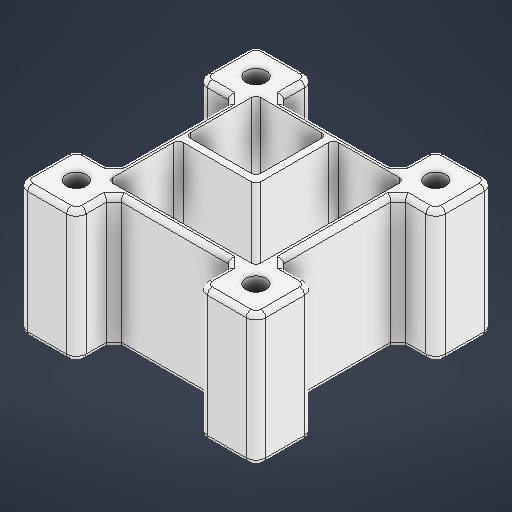
# Autodesk Inventor part: SemillasyAgua
Saved by Autodesk Inventor 2026.2 (Build 302298000, 298)
## iProperties
Created: 2025-11-15
Part Number: SemillasyAgua
Material: PLA
Document SubType Name: Modeling
Designer: vickh
Density: 1.3 g/cm^3
Appearance: Genérico
Mass: 211.053 g
Surface Area: 621.893 cm^2
Volume: 162.348 cm^3
Author: vickh
## iProperties of the stored document SemillasyAgua_3DPrint.ipt
Created: 2025-11-18
Part Number: SemillasyAgua_3DPrint
Material: Genérico
Document SubType Name: Modeling
Designer: usuario
Density: 1 g/cm^3
Appearance: Valor por defecto
Author: usuario
Autodesk Inventor part; units mm, degrees
ref_plane "YZ Plane" through (0, 0, 0) normal (1, 0, 0) x (0, 1, 0)
ref_plane "XZ Plane" through (0, 0, 0) normal (0, 1, 0) x (-1, 0, 0)
ref_plane "XY Plane" through (0, 0, 0) normal (0, 0, 1) x (1, 0, 0)
sketch "Boceto1" plane through (0, 0, 0) normal (0, 1, 0) x (-1, 0, 0)
  line L0 (25, 33.5) -> (-25, 33.5)
  line L1 (33.5, -25) -> (33.5, 25)
  circle A0 centre (0, 0) radius 5 construction
  line L2 (-33.5, 25) -> (-33.5, -25)
  line L3 (-25, -33.5) -> (25, -33.5)
  line L4 (-25, -49) -> (-25, -33.5)
  line L5 (-33.5, -25) -> (-49, -25)
  line L6 (-49, -25) -> (-49, -49)
  line L7 (-49, -49) -> (-25, -49)
  line L8 (-49, 25) -> (-33.5, 25)
  line L9 (-49, 49) -> (-49, 25)
  line L10 (-25, 49) -> (-49, 49)
  line L11 (-25, 33.5) -> (-25, 49)
  line L12 (33.5, 25) -> (49, 25)
  circle A1 centre (37, 37) radius 4.15
  line L13 (49, 25) -> (49, 49)
  line L14 (49, 49) -> (25, 49)
  line L15 (25, 49) -> (25, 33.5)
  line L16 (49, -49) -> (49, -25)
  line L17 (49, -25) -> (33.5, -25)
  line L18 (25, -49) -> (49, -49)
  line L19 (25, -33.5) -> (25, -49)
  line L20 (49, -49) -> (-49, -49) construction
  line L21 (-49, -49) -> (-49, 49)
  line L22 (-49, 49) -> (49, 49) construction
  line L23 (49, 49) -> (49, -49) construction
  line L24 (49, -49) -> (15.5795, -49) construction
  line L25 (49, -27.4055) -> (49, -49) construction
  line L26 (0, -49) -> (0, 49) construction
  line L27 (49, 0) -> (-49, 0) construction
  line L28 (49, 49) -> (25, 49) construction
  line L29 (25, 49) -> (25, 25) construction
  line L30 (25, 25) -> (49, 25) construction
  line L31 (49, 25) -> (49, 49) construction
  line L32 (49, 49) -> (25, 25) construction
  line L33 (49, 25) -> (25, 49) construction
  circle A2 centre (-37, 37) radius 4.15
  circle A3 centre (-37, -37) radius 4.15
  circle A4 centre (37, -37) radius 4.15
  line L34 (30.5, 30.5) -> (-30.5, 30.5)
  line L35 (-30.5, 30.5) -> (-30.5, -30.5)
  line L36 (-30.5, -30.5) -> (30.5, -30.5)
  line L37 (30.5, -30.5) -> (30.5, 30.5)
  line L38 (30.5, 30.5) -> (-30.5, -30.5) construction
  line L39 (-30.5, 30.5) -> (30.5, -30.5) construction
  circle A5 centre (0, 0) radius 2.5 construction
  point P0 (33.5, 0)
  point P1 (0, -33.5)
  point P2 (0, 33.5)
  point P3 (-33.5, 0)
  dimension "d2" = 33.5
  dimension "d3" = 33.5
  dimension "d4" = 8.3
  dimension "d5" = 49
  dimension "d6" = 49
  dimension "d7" = 98
  dimension "d8" = 98
  dimension "d9" = 15.5
  dimension "d10" = 15.5
  dimension "d11" = 15.5
  dimension "d12" = 15.5
  dimension "d13" = 50
  dimension "d14" = 50
  dimension "d15" = 15.5
  dimension "d16" = 15.5
  dimension "d17" = 15.5
  dimension "d18" = 50
  dimension "d19" = 25
  dimension "d20" = 25
  dimension "d21" = 25
  dimension "d22" = 25
  dimension "d23" = 10
  dimension "d24" = 8.5
  dimension "d25" = 8.5
  dimension "d26" = 24
  dimension "d27" = 15.5
  dimension "d28" = 24
  dimension "d29" = 8.5
  dimension "d30" = 24
  dimension "d31" = 24
  dimension "d32" = 360
  dimension "d33" = 3
  dimension "d34" = 5
  dimension "d35" = 3
  constraints: 80 end point, 11 midpoint, 7 horizontal, 7 vertical, 6 centre point, 6 parallel, 4 coincident, 3 perpendicular, 3 point on line, 9 other
  measures "d2" distance of point (0, 0) point (33.5, 0)
  measures "d3" distance from line of point (0, 0) L2
  measures "d4" diameter of A1
  measures "d5" distance of point (0, 0) L27.end
  measures "d6" distance from line of L20 point (0, 0)
  measures "d7" distance of L23.end L21.start
  measures "d8" distance of L21.start L21.end
  measures "d9" distance between parallel lines of L22 L0
  measures "d10" distance between parallel lines of L23 L1
  measures "d11" distance between parallel lines of L20 L3
  measures "d12" distance of L2.end L5.end
  measures "d13" distance of L4.end L19.start
  measures "d14" distance of L15.end L0.end
  measures "d15" distance of L14.end L15.end
  measures "d16" distance of L0.end L11.end
  measures "d17" distance of L8.start L2.start
  measures "d18" distance of L2.start L2.end
  measures "d19" distance from line of point (0, 0) L5
  measures "d20" distance from line of L17 point (0, 0)
  measures "d21" distance from line of point (0, 0) L12
  measures "d22" distance from line of point (0, 0) L8
  measures "d23" diameter of A0
  measures "d24" horizontal distance of L2.end L4.end
  measures "d25" distance from line of L11 L2.start
  measures "d26" distance of L12.end L13.end
  measures "d27" distance of L4.start L4.end
  measures "d28" distance of L13.end L14.end
  measures "d29" horizontal distance of L17.end L19.start
  measures "d30" distance of L30.end L30.start
  measures "d31" distance of L30.start L28.end
  measures "d33" distance between parallel lines of L36 L3
  measures "d34" diameter of A5
  measures "d35" distance between parallel lines of L1 L37
extrude "Extrusión1" add sketch "Boceto1" along normal blind 54 contours L15 L14 L13 L12 L1 L17 L16 L18 L19 L3 L4 L7 L6 L5 L2 L8 L9 L10 L11 L0
extrude "Extrusión2" add sketch "Boceto1" along normal blind 4 contours L37 L36 L35 L34
sketch "Boceto2" plane through (0, 4, 0) normal (0, 1, 0) x (1, 0, 0)
  line L0 (-1.5, -30.5) -> (-1.5, 30.5)
  line L1 (-1.5, 30.5) -> (1.5, 30.5)
  line L2 (1.5, 30.5) -> (1.5, -30.5)
  line L3 (1.5, -30.5) -> (-1.5, -30.5)
  line L4 (-1.5, -30.5) -> (1.5, 30.5) construction
  line L5 (-1.5, 30.5) -> (1.5, -30.5) construction
  line L6 (30.5, 30.5) -> (30.5, -30.5) projected
  line L7 (-30.5, 30.5) -> (30.5, 30.5) projected
  line L8 (30.5, -1.5) -> (-30.5, -1.5)
  line L9 (-30.5, -1.5) -> (-30.5, 1.5)
  line L10 (-30.5, 1.5) -> (30.5, 1.5)
  line L11 (30.5, 1.5) -> (30.5, -1.5)
  line L12 (30.5, -1.5) -> (-30.5, 1.5) construction
  line L13 (-30.5, -1.5) -> (30.5, 1.5) construction
  line L14 (-30.5, -30.5) -> (-30.5, 30.5) projected
  point P0 (0, 0)
  point P1 (30.5, 0)
  point P2 (-1.5, 1.5)
  point P3 (-1.5, -1.5)
  point P4 (1.5, 1.5)
  point P5 (1.5, -1.5)
  dimension "d40" = 3
  dimension "d45" = 3
  constraints: 24 end point, 5 midpoint, 4 parallel, 3 perpendicular, 2 collinear, 1 vertical
  measures "d40" distance of L0.end L1.end
  measures "d45" distance of L8.end L9.end
extrude "Extrusión3" add sketch "Boceto2" along normal up to surface (50 mm away) contours L8 L9 L10 L0 | L0 L10 L2 L8 | L0 L1 L2 L10
fillet "Empalme1" radius 4 12 edges at (49, 27, 49) (49, 27, 25) (49, 27, -25) (49, 27, -49) (25, 27, -49) (-25, 27, -49) (-49, 27, -49) (-49, 27, -25) (-49, 27, 25) (-49, 27, 49) (-25, 27, 49) (25, 27, 49)
chamfer "Chaflán1" distance 3 angle 45 8 edges at (-33.5, 27, 25) (-33.5, 27, -25) (-25, 27, -33.5) (25, 27, -33.5) (33.5, 27, -25) (33.5, 27, 25) (25, 27, 33.5) (-25, 27, 33.5)
sketch "Boceto3" plane through (1.5, 4, 1.5) normal (1, 0, 0) x (0, 0, -1)
  point P0 (1.5, -4)
fillet "Empalme2" radius 2 12 edges at (1.5, 29, 1.5) (-30.5, 29, 1.5) (1.5, 29, -30.5) (30.5, 29, -30.5) (30.5, 29, 30.5) (-30.5, 29, 30.5) (-14.5, 4, 1.5) (1.5, 4, -14.5) (16, 4, -30.5) (30.5, 4, 0) (0, 4, 30.5) (-30.5, 4, 16)
fillet "Empalme3" radius 2 80 edges at (26.1716, 0, 47.8284) (25, 0, 40.75) (23.5, 0, 35) (0, 0, 33.5) (-23.5, 0, 35) (-25, 0, 40.75) (-26.1716, 0, 47.8284) (-37, 0, 49) (-47.8284, 0, 47.8284) (-49, 0, 37) (-47.8284, 0, 26.1716) (-40.75, 0, 25) (-35, 0, 23.5) (-33.5, 0, 0) (-35, 0, -23.5) (-40.75, 0, -25) (-47.8284, 0, -26.1716) (-49, 0, -37) (-47.8284, 0, -47.8284) (-37, 0, -49) (-26.1716, 0, -47.8284) (-25, 0, -40.75) (-23.5, 0, -35) (0, 0, -33.5) (23.5, 0, -35) (25, 0, -40.75) (26.1716, 0, -47.8284) (37, 0, -49) (47.8284, 0, -47.8284) (49, 0, -37) (47.8284, 0, -26.1716) (40.75, 0, -25) (35, 0, -23.5) (33.5, 0, 0) (35, 0, 23.5) (40.75, 0, 25) (47.8284, 0, 26.1716) (49, 0, 37) (47.8284, 0, 47.8284) (37, 0, 49) (26.1716, 54, 47.8284) (37, 54, 49) (47.8284, 54, 47.8284) (49, 54, 37) (47.8284, 54, 26.1716) (40.75, 54, 25) (35, 54, 23.5) (33.5, 54, 0) (35, 54, -23.5) (40.75, 54, -25) (47.8284, 54, -26.1716) (49, 54, -37) (47.8284, 54, -47.8284) (37, 54, -49) (26.1716, 54, -47.8284) (25, 54, -40.75) (23.5, 54, -35) (0, 54, -33.5) (-23.5, 54, -35) (-25, 54, -40.75) (-26.1716, 54, -47.8284) (-37, 54, -49) (-47.8284, 54, -47.8284) (-49, 54, -37) (-47.8284, 54, -26.1716) (-40.75, 54, -25) (-35, 54, -23.5) (-33.5, 54, 0) (-35, 54, 23.5) (-40.75, 54, 25) (-47.8284, 54, 26.1716) (-49, 54, 37) (-47.8284, 54, 47.8284) (-37, 54, 49) (-26.1716, 54, 47.8284) (-25, 54, 40.75) (-23.5, 54, 35) (0, 54, 33.5) (23.5, 54, 35) (25, 54, 40.75)
fillet "Empalme4" radius 2 4 edges at (-30.5, 29, -30.5) (-1.5, 29, -30.5) (-1.5, 29, -1.5) (-30.5, 29, -1.5)
